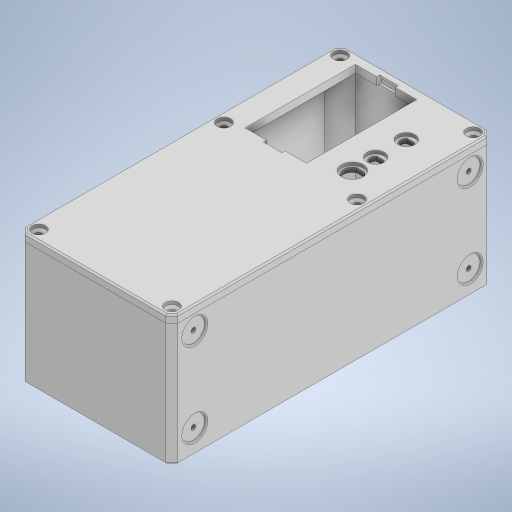
# Autodesk Inventor part: Light Beacon Box
Saved by Autodesk Inventor 2024 (Build 280153020, 153B)
## iProperties
Created: 2023-08-06
Part Number: Light Beacon Box
Material: Generic
Document SubType Name: Modeling
Designer: torban
Density: 1 g/cm^3
Appearance: Default
Author: torban
Autodesk Inventor part; units mm, degrees
ref_plane "YZ Plane" through (0, 0, 0) normal (1, 0, 0) x (0, 1, 0)
ref_plane "XZ Plane" through (0, 0, 0) normal (0, 1, 0) x (-1, 0, 0)
ref_plane "XY Plane" through (0, 0, 0) normal (0, 0, 1) x (1, 0, 0)
sketch "Sketch1" plane through (0, 0, 0) normal (0, 1, 0) x (-1, 0, 0)
  line L0 (0, 0) -> (90, 0)
  line L1 (90, 0) -> (90, -120)
  line L2 (90, -120) -> (0, -120)
  line L3 (0, -120) -> (0, 0)
  line L4 (90, -120) -> (0, -120)
  line L5 (0, -120) -> (0, -200)
  line L6 (0, -200) -> (90, -200)
  line L7 (90, -200) -> (90, -120)
  line L8 (95, -125) -> (95, 5)
  line L9 (95, 5) -> (-5, 5)
  line L10 (-5, 5) -> (-5, -125)
  line L11 (-5, -125) -> (95, -125)
  line L12 (95, -115) -> (-5, -115)
  line L13 (-5, -115) -> (-5, -205)
  line L14 (-5, -205) -> (95, -205)
  line L15 (95, -205) -> (95, -115)
  point P0 (0, -125)
  point P1 (90, -125)
  dimension "d0" = 120
  dimension "d1" = 90
  dimension "d2" = 90
  dimension "d3" = 80
  dimension "d4" = 5
  dimension "d5" = 5
  constraints: 32 end point, 8 parallel, 4 perpendicular, 2 horizontal, 6 other
  measures "d0" distance of L0.end L1.end
  measures "d1" distance of L1.end L2.end
  measures "d2" distance of L6.end L5.end
  measures "d3" distance of L6.end L1.end
  measures "d4" distance between parallel lines of L1 L8
  measures "d5" distance between parallel lines of L7 L15
extrude "Extrusion1" add sketch "Sketch1" along normal blind 75 contours L3 L12 L10 L9 L8 L1 L0 | L3 L5 L11 L10 L12 | L12 L8 L11 L7 L1 | L2 L7 L11 L5 | L5 L6 L7 L11 L15 L14 L13
sketch "Sketch3" plane through (0, 0, 0) normal (0, -1, 0) x (1, 0, 0)
  line L0 (0, -200) -> (0, -125) projected
  line L1 (0, -125) -> (-90, -125) projected
  line L2 (-90, -125) -> (-90, -200) projected
  line L3 (-90, -200) -> (0, -200) projected
  line L4 (-90, -120) -> (0, -120) projected
  line L5 (0, -120) -> (0, 0) projected
  line L6 (0, 0) -> (-90, 0) projected
  line L7 (-90, 0) -> (-90, -120) projected
  line L8 (-95, 5) -> (5, 5) projected
  line L9 (5, 5) -> (5, -205) projected
  line L10 (5, -205) -> (-95, -205) projected
  line L11 (-95, -205) -> (-95, 5) projected
extrude "Extrusion2" add sketch "Sketch3" along normal blind 5 contours L3 L2 L1 L0 | L7 L6 L5 L4 | L8 L9 L10 L11
sketch "Sketch4" plane through (-90, 75, -120) normal (0, 0, 1) x (1, 0, 0)
  line L0 (95, -80) -> (-5, -80) projected
  line L1 (-5, -80) -> (-5, 0) projected
  line L2 (-5, 0) -> (0, 0) projected
  line L3 (0, -75) -> (0, 0) projected
  line L4 (0, -75) -> (90, -75) projected
  line L5 (90, 0) -> (90, -75) projected
  line L6 (0, 0) -> (90, 0) projected
  line L7 (95, 0) -> (95, -80) projected
  line L8 (90, 0) -> (95, 0) projected
  line L9 (0, -55) -> (90, -55)
  line L10 (90, -75) -> (90, 0) projected
  line L11 (0, -55) -> (20, -55)
  line L12 (20, -55) -> (20, 0)
  line L13 (90, -55) -> (70, -55)
  line L14 (70, -55) -> (70, 0)
  circle A0 centre (20, -55) radius 5
  circle A1 centre (70, -55) radius 5
  dimension "d10" = 20
  dimension "d11" = 20
  dimension "d12" = 20
  dimension "d13" = 10
  dimension "d14" = 10
  constraints: 10 end point, 6 point on line, 3 perpendicular, 2 centre point, 2 coincident
  measures "d10" distance between parallel lines of L4 L9
  measures "d11" distance of L9.start L11.end
  measures "d12" distance of L9.end L13.end
  measures "d13" diameter of A0
  measures "d14" diameter of A1
extrude "Extrusion3" cut sketch "Sketch4" against normal up to surface (5 mm away) contours A1 L9 | L9 L14 A1 | L14 L9 A1 | A0 L12 L9 | L9 A0 | A0 L9 L12
chamfer "Chamfer1" distance 10 angle 45 8 edges at (-90, 37.5, -120) (-90, 37.5, -200) (-90, 37.5, 0) (0, 37.5, 0) (0, 37.5, -120) (0, 37.5, -200) (0, 37.5, -125) (-90, 37.5, -125)
sketch "Sketch5" plane through (0, 75, 0) normal (0, 1, 0) x (1, 0, 0)
  line L0 (-10, 125) -> (0, 135) projected
  line L1 (0, 135) -> (0, 190) projected
  line L2 (0, 190) -> (-10, 200) projected
  line L3 (-10, 200) -> (-80, 200) projected
  line L4 (-80, 200) -> (-90, 190) projected
  line L5 (-90, 190) -> (-90, 135) projected
  line L6 (-90, 135) -> (-80, 125) projected
  line L7 (-80, 125) -> (-10, 125) projected
  line L8 (-10, 0) -> (0, 10) projected
  line L9 (0, 10) -> (0, 110) projected
  line L10 (0, 110) -> (-10, 120) projected
  line L11 (-10, 120) -> (-80, 120) projected
  line L12 (-80, 120) -> (-90, 110) projected
  line L13 (-90, 110) -> (-90, 10) projected
  line L14 (-90, 10) -> (-80, 0) projected
  line L15 (-80, 0) -> (-10, 0) projected
  line L16 (5, -5) -> (-95, -5) projected
  line L17 (-95, -5) -> (-95, 205) projected
  line L18 (-95, 205) -> (5, 205) projected
  line L19 (5, 205) -> (5, -5) projected
  line L20 (-88.5, 198.5) -> (-88.5, 1.5)
  line L21 (-88.5, 1.5) -> (-1.5, 1.5)
  line L22 (-1.5, 1.5) -> (-1.5, 198.5)
  line L23 (-1.5, 198.5) -> (-88.5, 198.5)
  line L24 (-75, 120) -> (-75, 125) projected
  line L25 (-75, 122.5) -> (-88.5, 122.5)
  line L26 (-75, 122.5) -> (-1.5, 122.5)
  point P0 (0, 0)
  dimension "d20" = 6.5
  dimension "d80" = 0
  constraints: 12 end point, 5 coincident, 4 point on line, 1 perpendicular, 6 other
  measures "d20" distance between parallel lines of L17 L20
  measures "d80" distance from line of L23 point (-1.5, 198.5)
hole "Hole1" at (-88.5, 75, -1.5) at (-88.5, 75, -198.5) at (-1.5, 75, -198.5) at (-1.5, 75, -1.5) at (-88.5, 75, -122.5) at (-1.5, 75, -122.5) direction (0, -1, 0) diameter 4.69 depth 20 tip angle 118
chamfer "Chamfer2" distance 4 angle 45 4 edges at (-95, 35, 5) (5, 35, 5) (-95, 35, -205) (5, 35, -205)
sketch "Sketch6" plane through (0, 75, 0) normal (0, 1, 0) x (1, 0, 0)
  line L0 (-91, -5) -> (-95, -1) projected
  line L1 (-95, -1) -> (-95, 201) projected
  line L2 (-95, 201) -> (-91, 205) projected
  line L3 (-91, 205) -> (1, 205) projected
  line L4 (1, 205) -> (5, 201) projected
  line L5 (5, 201) -> (5, -1) projected
  line L6 (5, -1) -> (1, -5) projected
  line L7 (1, -5) -> (-91, -5) projected
  line L8 (-80, 125) -> (-10, 125) projected
  line L9 (-10, 125) -> (0, 135) projected
  line L10 (0, 135) -> (0, 190) projected
  line L11 (0, 190) -> (-10, 200) projected
  line L12 (-10, 200) -> (-80, 200) projected
  line L13 (-80, 200) -> (-90, 190) projected
  line L14 (-90, 190) -> (-90, 135) projected
  line L15 (-90, 135) -> (-80, 125) projected
  line L16 (0, 10) -> (0, 110) projected
  line L17 (0, 110) -> (-10, 120) projected
  line L18 (-10, 120) -> (-80, 120) projected
  line L19 (-80, 120) -> (-90, 110) projected
  line L20 (-90, 110) -> (-90, 10) projected
  line L21 (-90, 10) -> (-80, 0) projected
  line L22 (-80, 0) -> (-10, 0) projected
  line L23 (-10, 0) -> (0, 10) projected
  circle A0 centre (-88.5, 1.5) radius 2.345 projected
  circle A1 centre (-88.5, 198.5) radius 2.345 projected
  circle A2 centre (-1.5, 198.5) radius 2.345 projected
  circle A3 centre (-1.5, 1.5) radius 2.345 projected
  circle A4 centre (-88.5, 122.5) radius 2.345 projected
  circle A5 centre (-1.5, 122.5) radius 2.345 projected
  point P0 (0, 0)
extrude "Extrusion4" add sketch "Sketch6" along normal blind 5 separate body
sketch "Sketch7" plane through (0, 80, 0) normal (0, 1, 0) x (1, 0, 0)
  line L0 (-80, 125) -> (-10, 125) projected
  line L1 (-10, 125) -> (0, 135) projected
  line L2 (0, 135) -> (0, 190) projected
  line L3 (0, 190) -> (-10, 200) projected
  line L4 (-10, 200) -> (-80, 200) projected
  line L5 (-80, 200) -> (-90, 190) projected
  line L6 (-90, 190) -> (-90, 135) projected
  line L7 (-90, 135) -> (-80, 125) projected
  line L8 (0, 10) -> (0, 110) projected
  line L9 (0, 110) -> (-10, 120) projected
  line L10 (-10, 120) -> (-80, 120) projected
  line L11 (-80, 120) -> (-90, 110) projected
  line L12 (-90, 110) -> (-90, 10) projected
  line L13 (-90, 10) -> (-80, 0) projected
  line L14 (-80, 0) -> (-10, 0) projected
  line L15 (-10, 0) -> (0, 10) projected
  circle A0 centre (-88.5, 1.5) radius 2.345 projected
  circle A1 centre (-88.5, 198.5) radius 2.345 projected
  circle A2 centre (-1.5, 198.5) radius 2.345 projected
  circle A3 centre (-1.5, 1.5) radius 2.345 projected
  circle A4 centre (-1.5, 122.5) radius 2.345 projected
  circle A5 centre (-88.5, 122.5) radius 2.345 projected
  line L16 (1, -5) -> (-91, -5) projected
  line L17 (-91, -5) -> (-95, -1) projected
  line L18 (-95, -1) -> (-95, 201) projected
  line L19 (-95, 201) -> (-91, 205) projected
  line L20 (-91, 205) -> (1, 205) projected
  line L21 (1, 205) -> (5, 201) projected
  line L22 (5, 201) -> (5, -1) projected
  line L23 (5, -1) -> (1, -5) projected
  line L24 (-78.5, 126.5) -> (-38.5, 126.5)
  line L25 (-38.5, 126.5) -> (-38.5, 198.5)
  line L26 (-38.5, 198.5) -> (-78.5, 198.5)
  line L27 (-78.5, 198.5) -> (-78.5, 126.5)
  point P0 (0, 0)
  point P1 (-58.5, 198.5)
  dimension "d33" = 72
  dimension "d35" = 40
  dimension "d40" = 1.5
  dimension "d41" = 1.5
  constraints: 8 end point, 2 parallel, 1 horizontal, 1 midpoint, 1 perpendicular
  measures "d33" distance between parallel lines of L26 L24
  measures "d35" distance of L25.end L26.end
  measures "d40" distance from line of L4.end L27
  measures "d41" distance between parallel lines of L0 L24
extrude "Extrusion5" add sketch "Sketch7" against normal blind 5 contours L7 L6 L5 L4 L3 L2 L1 L0 | L15 L14 L13 L12 L11 L10 L9 L8 | L16 L17 L18 L19 L20 L21 L22 L23 bodies 2
sketch "Sketch8" plane through (0, 80, 0) normal (0, 1, 0) x (1, 0, 0)
  line L0 (-38.5, 198.5) -> (-78.5, 198.5) projected
  line L1 (-78.5, 198.5) -> (-78.5, 126.5) projected
  line L2 (-78.5, 126.5) -> (-38.5, 126.5) projected
  line L3 (-38.5, 126.5) -> (-38.5, 198.5) projected
  circle A0 centre (-88.5, 1.5) radius 2.345 projected
  circle A1 centre (-88.5, 198.5) radius 2.345 projected
  circle A2 centre (-1.5, 198.5) radius 2.345 projected
  circle A3 centre (-1.5, 1.5) radius 2.345 projected
  circle A4 centre (-1.5, 122.5) radius 2.345 projected
  circle A5 centre (-88.5, 122.5) radius 2.345 projected
  line L4 (1, -5) -> (-91, -5) projected
  line L5 (-91, -5) -> (-95, -1) projected
  line L6 (-95, -1) -> (-95, 201) projected
  line L7 (-95, 201) -> (-91, 205) projected
  line L8 (-91, 205) -> (1, 205) projected
  line L9 (1, 205) -> (5, 201) projected
  line L10 (5, 201) -> (5, -1) projected
  line L11 (5, -1) -> (1, -5) projected
  line L12 (-64.5, 124.5) -> (-52.5, 124.5)
  line L13 (-52.5, 124.5) -> (-52.5, 200.5)
  line L14 (-52.5, 200.5) -> (-64.5, 200.5)
  line L15 (-64.5, 200.5) -> (-64.5, 124.5)
  point P0 (0, 0)
  point P1 (-64.5, 198.5)
  point P2 (-52.5, 198.5)
  point P3 (-52.5, 126.5)
  point P4 (-64.5, 126.5)
  dimension "d44" = 12
  dimension "d46" = 14
  dimension "d47" = 14
  dimension "d48" = 76
  dimension "d49" = 2
  constraints: 8 end point, 2 parallel, 1 horizontal, 1 perpendicular
  measures "d44" distance of L12.start L12.end
  measures "d46" distance between parallel lines of L3 L13
  measures "d47" distance between parallel lines of L1 L15
  measures "d48" distance between parallel lines of L14 L12
  measures "d49" distance between parallel lines of L2 L12
extrude "Extrusion6" cut sketch "Sketch8" against normal blind 5 contours L0 L15 L14 L13 | L13 L12 L15 L2 bodies 2
sketch "Sketch9" plane through (0, 75, 0) normal (0, 1, 0) x (1, 0, 0)
  line L0 (-91, -5) -> (-95, -1) projected
  line L1 (-95, -1) -> (-95, 201) projected
  line L2 (-95, 201) -> (-91, 205) projected
  line L3 (-91, 205) -> (1, 205) projected
  line L4 (1, 205) -> (5, 201) projected
  line L5 (5, 201) -> (5, -1) projected
  line L6 (5, -1) -> (1, -5) projected
  line L7 (1, -5) -> (-91, -5) projected
  line L8 (-80, 125) -> (-10, 125) projected
  line L9 (-10, 125) -> (0, 135) projected
  line L10 (0, 135) -> (0, 190) projected
  line L11 (0, 190) -> (-10, 200) projected
  line L12 (-10, 200) -> (-80, 200) projected
  line L13 (-80, 200) -> (-90, 190) projected
  line L14 (-90, 190) -> (-90, 135) projected
  line L15 (-90, 135) -> (-80, 125) projected
  line L16 (0, 10) -> (0, 110) projected
  line L17 (0, 110) -> (-10, 120) projected
  line L18 (-10, 120) -> (-80, 120) projected
  line L19 (-80, 120) -> (-90, 110) projected
  line L20 (-90, 110) -> (-90, 10) projected
  line L21 (-90, 10) -> (-80, 0) projected
  line L22 (-80, 0) -> (-10, 0) projected
  line L23 (-10, 0) -> (0, 10) projected
  circle A0 centre (-88.5, 1.5) radius 2.345 projected
  circle A1 centre (-88.5, 198.5) radius 2.345 projected
  circle A2 centre (-1.5, 198.5) radius 2.345 projected
  circle A3 centre (-1.5, 1.5) radius 2.345 projected
  circle A4 centre (-88.5, 122.5) radius 2.345 projected
  circle A5 centre (-1.5, 122.5) radius 2.345 projected
  line L24 (-64.5, 126.5) -> (-64.5, 124.5) projected
  line L25 (-64.5, 124.5) -> (-52.5, 124.5) projected
  line L26 (-52.5, 124.5) -> (-52.5, 126.5) projected
  line L27 (-52.5, 126.5) -> (-38.5, 126.5) projected
  line L28 (-38.5, 126.5) -> (-38.5, 198.5) projected
  line L29 (-38.5, 198.5) -> (-52.5, 198.5) projected
  line L30 (-52.5, 198.5) -> (-52.5, 200.5) projected
  line L31 (-52.5, 200.5) -> (-64.5, 200.5) projected
  line L32 (-64.5, 200.5) -> (-64.5, 198.5) projected
  line L33 (-64.5, 198.5) -> (-78.5, 198.5) projected
  line L34 (-78.5, 198.5) -> (-78.5, 126.5) projected
  line L35 (-78.5, 126.5) -> (-64.5, 126.5) projected
  circle A6 centre (-88.5, 1.5) radius 2.345 projected
  circle A7 centre (-88.5, 198.5) radius 2.345 projected
  circle A8 centre (-1.5, 198.5) radius 2.345 projected
  circle A9 centre (-1.5, 1.5) radius 2.345 projected
  circle A10 centre (-1.5, 122.5) radius 2.345 projected
  circle A11 centre (-88.5, 122.5) radius 2.345 projected
  line L36 (5, -1) -> (1, -5) projected
  line L37 (1, -5) -> (-91, -5) projected
  line L38 (-91, -5) -> (-95, -1) projected
  line L39 (-95, -1) -> (-95, 201) projected
  line L40 (-95, 201) -> (-91, 205) projected
  line L41 (-91, 205) -> (1, 205) projected
  line L42 (1, 205) -> (5, 201) projected
  line L43 (5, 201) -> (5, -1) projected
  line L44 (-64.5, 126.5) -> (-52.5, 126.5)
  line L45 (-52.5, 126.5) -> (-52.5, 123.5)
  line L46 (-52.5, 123.5) -> (-64.5, 123.5)
  line L47 (-64.5, 123.5) -> (-64.5, 126.5)
  line L48 (-64.5, 198.5) -> (-52.5, 198.5)
  line L49 (-52.5, 198.5) -> (-52.5, 201.5)
  line L50 (-52.5, 201.5) -> (-64.5, 201.5)
  line L51 (-64.5, 201.5) -> (-64.5, 198.5)
  point P0 (0, 0)
  point P1 (-52.5, 199.5)
  point P2 (-52.5, 200)
  dimension "d52" = 78
  dimension "d53" = 1
  dimension "d54" = 1
  dimension "d55" = 0
  dimension "d56" = 0
  constraints: 16 end point, 4 parallel, 4 point on line, 2 horizontal, 2 midpoint, 2 perpendicular
  measures "d52" distance between parallel lines of L50 L46
  measures "d53" distance between parallel lines of L25 L46
  measures "d54" distance between parallel lines of L50 L31
  measures "d55" distance between parallel lines of L32 L51
  measures "d56" horizontal distance of point (-52.5, 199.5) point (-52.5, 200)
extrude "Extrusion7" cut sketch "Sketch9" along normal blind 3.5 contours L25 L45 L46 L47 | L51 L50 L49 L31 bodies 2
sketch "Sketch10" plane through (0, 80, 0) normal (0, 1, 0) x (1, 0, 0)
  line L0 (-52.5, 200.5) -> (-52.5, 198.5) projected
  line L1 (-52.5, 198.5) -> (-38.5, 198.5) projected
  line L2 (-38.5, 198.5) -> (-38.5, 126.5) projected
  line L3 (-38.5, 126.5) -> (-52.5, 126.5) projected
  line L4 (-52.5, 126.5) -> (-52.5, 124.5) projected
  line L5 (-52.5, 124.5) -> (-64.5, 124.5) projected
  line L6 (-64.5, 124.5) -> (-64.5, 126.5) projected
  line L7 (-64.5, 126.5) -> (-78.5, 126.5) projected
  line L8 (-78.5, 126.5) -> (-78.5, 198.5) projected
  line L9 (-78.5, 198.5) -> (-64.5, 198.5) projected
  line L10 (-64.5, 198.5) -> (-64.5, 200.5) projected
  line L11 (-64.5, 200.5) -> (-52.5, 200.5) projected
  line L12 (1, -5) -> (5, -1) projected
  line L13 (5, -1) -> (5, 201) projected
  line L14 (5, 201) -> (1, 205) projected
  line L15 (1, 205) -> (-91, 205) projected
  line L16 (-91, 205) -> (-95, 201) projected
  line L17 (-95, 201) -> (-95, -1) projected
  line L18 (-95, -1) -> (-91, -5) projected
  line L19 (-91, -5) -> (1, -5) projected
  circle A0 centre (-88.5, 122.5) radius 2.345 projected
  circle A1 centre (-1.5, 122.5) radius 2.345 projected
  circle A2 centre (-1.5, 1.5) radius 2.345 projected
  circle A3 centre (-1.5, 198.5) radius 2.345 projected
  circle A4 centre (-88.5, 198.5) radius 2.345 projected
  circle A5 centre (-88.5, 1.5) radius 2.345 projected
  line L20 (0, 190) -> (0, 135) projected
  line L21 (-38.5, 126.5) -> (-38.5, 198.5) projected
  line L22 (-38.5, 162.5) -> (0, 162.5)
  line L23 (-19.25, 162.5) -> (-19.25, 172.5)
  line L24 (-19.25, 172.5) -> (-19.25, 152.5)
  circle A6 centre (-19.25, 172.5) radius 3.875
  circle A7 centre (-19.25, 152.5) radius 3.875
  line L25 (-21.7027, 149.5) -> (-16.7973, 149.5)
  line L26 (-16.7973, 149.5) -> (-16.7973, 155.5)
  line L27 (-16.7973, 155.5) -> (-21.7027, 155.5)
  line L28 (-21.7027, 155.5) -> (-21.7027, 149.5)
  line L29 (-21.7027, 149.5) -> (-16.7973, 155.5) construction
  line L30 (-16.7973, 149.5) -> (-21.7027, 155.5) construction
  line L31 (-21.7027, 175.5) -> (-16.7973, 175.5)
  line L32 (-16.7973, 175.5) -> (-16.7973, 169.5)
  line L33 (-16.7973, 169.5) -> (-21.7027, 169.5)
  line L34 (-21.7027, 169.5) -> (-21.7027, 175.5)
  line L35 (-21.7027, 175.5) -> (-16.7973, 169.5) construction
  line L36 (-16.7973, 175.5) -> (-21.7027, 169.5) construction
  point P0 (0, 0)
  dimension "d61" = 7.75
  dimension "d62" = 7.75
  dimension "d59" = 10
  dimension "d60" = 20
  dimension "d63" = 6
  constraints: 30 end point, 7 midpoint, 4 parallel, 3 perpendicular, 2 coincident, 2 horizontal, 2 point on line, 6 other
  measures "d59" distance of L23.start L23.end
  measures "d60" distance of L23.end L24.end
  measures "d63" distance of L26.end L25.end
extrude "Extrusion8" cut sketch "Sketch10" against normal blind 5 contours L33 L34 L31 L32 | A6 L34 | L32 A6 | L27 L26 L25 L28 | A7 L26 | L28 A7 bodies 2
sketch "Sketch11" plane through (0, 80, 0) normal (0, 1, 0) x (1, 0, 0)
  arc A0 (-16.7973, 169.5) -> (-16.7973, 175.5) centre (-19.25, 172.5) ccw projected
  line L0 (-16.7973, 169.5) -> (-21.7027, 169.5) projected
  arc A1 (-21.7027, 175.5) -> (-21.7027, 169.5) centre (-19.25, 172.5) ccw projected
  line L1 (-21.7027, 175.5) -> (-16.7973, 175.5) projected
  arc A2 (-16.7973, 149.5) -> (-16.7973, 155.5) centre (-19.25, 152.5) ccw projected
  line L2 (-16.7973, 149.5) -> (-21.7027, 149.5) projected
  arc A3 (-21.7027, 155.5) -> (-21.7027, 149.5) centre (-19.25, 152.5) ccw projected
  line L3 (-21.7027, 155.5) -> (-16.7973, 155.5) projected
  line L4 (-52.5, 200.5) -> (-52.5, 198.5) projected
  line L5 (-52.5, 198.5) -> (-38.5, 198.5) projected
  line L6 (-38.5, 198.5) -> (-38.5, 126.5) projected
  line L7 (-38.5, 126.5) -> (-52.5, 126.5) projected
  line L8 (-52.5, 126.5) -> (-52.5, 124.5) projected
  line L9 (-52.5, 124.5) -> (-64.5, 124.5) projected
  line L10 (-64.5, 124.5) -> (-64.5, 126.5) projected
  line L11 (-64.5, 126.5) -> (-78.5, 126.5) projected
  line L12 (-78.5, 126.5) -> (-78.5, 198.5) projected
  line L13 (-78.5, 198.5) -> (-64.5, 198.5) projected
  line L14 (-64.5, 198.5) -> (-64.5, 200.5) projected
  line L15 (-64.5, 200.5) -> (-52.5, 200.5) projected
  line L16 (1, -5) -> (5, -1) projected
  line L17 (5, -1) -> (5, 201) projected
  line L18 (5, 201) -> (1, 205) projected
  line L19 (1, 205) -> (-91, 205) projected
  line L20 (-91, 205) -> (-95, 201) projected
  line L21 (-95, 201) -> (-95, -1) projected
  line L22 (-95, -1) -> (-91, -5) projected
  line L23 (-91, -5) -> (1, -5) projected
  circle A4 centre (-88.5, 122.5) radius 2.345 projected
  circle A5 centre (-1.5, 122.5) radius 2.345 projected
  circle A6 centre (-1.5, 1.5) radius 2.345 projected
  circle A7 centre (-1.5, 198.5) radius 2.345 projected
  circle A8 centre (-88.5, 198.5) radius 2.345 projected
  circle A9 centre (-88.5, 1.5) radius 2.345 projected
  point P0 (0, 0)
  point P1 (-1.5, 1.5)
  constraints: 5 coincident
hole "Hole3" at (-88.5, 80, -1.5) at (-88.5, 80, -122.5) at (-88.5, 80, -198.5) at (-1.5, 80, -198.5) at (-1.5, 80, -122.5) at (-1.5, 80, -1.5) direction (0, -1, 0) diameter 8.7 depth 2 tip angle 118 bodies 2
sketch "Sketch2" plane through (0, 0, -125) normal (0, 0, -1) x (-1, 0, 0)
  line L0 (-5, -5) -> (-5, 75) projected
  line L1 (-5, 75) -> (10, 75) projected
  line L2 (80, 75) -> (95, 75) projected
  line L3 (95, 75) -> (95, -5) projected
  line L4 (80, 0) -> (80, 75) projected
  line L5 (10, 75) -> (80, 75) projected
  line L6 (95, -5) -> (-5, -5) projected
  circle A0 centre (20, 20) radius 5 projected
  circle A1 centre (70, 20) radius 5 projected
  line L7 (95, 75) -> (64.5, 75) projected
  line L8 (64.5, 75) -> (64.5, 80) projected
  line L9 (64.5, 80) -> (84.9402, 80) projected
  line L10 (84.9402, 80) -> (84.9402, 78) projected
  line L11 (92.0598, 78) -> (92.0598, 80) projected
  line L12 (92.0598, 80) -> (95, 80) projected
  line L13 (95, 80) -> (95, 75) projected
  line L14 (52.5, 75) -> (-5, 75) projected
  line L15 (-5, 75) -> (-5, 80) projected
  line L16 (-5, 80) -> (-2.0598, 80) projected
  line L17 (-2.0598, 80) -> (-2.0598, 78) projected
  line L18 (5.0598, 78) -> (5.0598, 80) projected
  line L19 (5.0598, 80) -> (52.5, 80) projected
  line L20 (52.5, 80) -> (52.5, 75) projected
  line L21 (10, 0) -> (10, 75) projected
  line L22 (10, 0) -> (80, 0) projected
  constraints: 2 horizontal alignment
sketch "Sketch12" plane through (0, 80, 0) normal (0, 1, 0) x (1, 0, 0)
  line L0 (-90, 10) -> (-90, 110) projected
  circle A0 centre (-88.5, 1.5) radius 4.35 projected
  line L1 (-90, 10) -> (-80, 0) projected
  line L2 (-10, 0) -> (-80, 0) projected
  line L3 (-10, 0) -> (0, 10) projected
  line L4 (-38.5, 198.5) -> (-38.5, 126.5) projected
  line L5 (-38.5, 162.5) -> (0, 162.5)
  line L6 (0, 190) -> (0, 135) projected
  line L7 (-10, 125) -> (-80, 125) projected
  line L8 (-10, 125) -> (-80, 125) projected
  line L9 (-21.7027, 149.5) -> (-16.7973, 149.5) projected
  line L10 (-19.25, 149.5) -> (-19.25, 125)
  circle A1 centre (-19.25, 137.25) radius 5.8
  line L11 (-16.7847, 142.5) -> (-21.7153, 142.5)
  line L12 (-21.7153, 142.5) -> (-21.7153, 132)
  line L13 (-21.7153, 132) -> (-16.7847, 132)
  line L14 (-16.7847, 132) -> (-16.7847, 142.5)
  line L15 (-16.7847, 142.5) -> (-21.7153, 132) construction
  line L16 (-21.7153, 142.5) -> (-16.7847, 132) construction
  point P0 (0, 0)
  point P1 (-10, 120)
  dimension "d84" = 11.6
  dimension "d85" = 10.5
  constraints: 16 end point, 6 midpoint, 2 parallel, 2 perpendicular, 1 horizontal, 1 point on line, 3 other
  measures "d85" distance of L12.end L11.end
extrude "Extrusion9" cut sketch "Sketch12" against normal blind 5 contours L11 L14 L13 L10 | L10 L13 L12 L11 | A1 L14 | L12 A1 bodies 2
fillet "Fillet1" radius 2.5 4 edges at (-75, 20, -120) (-75, 20, -125) (-25, 20, -120) (-25, 20, -125)
sketch "Sketch13" plane through (0, 80, 0) normal (0, 1, 0) x (1, 0, 0)
  arc A0 (-21.7153, 142.5) -> (-21.7153, 132) centre (-19.25, 137.25) ccw projected
  line L0 (-21.7153, 142.5) -> (-16.7847, 142.5) projected
  arc A1 (-16.7847, 132) -> (-16.7847, 142.5) centre (-19.25, 137.25) ccw projected
  line L1 (-16.7847, 132) -> (-21.7153, 132) projected
  circle A2 centre (-1.5, 1.5) radius 4.35 projected
  circle A3 centre (-1.5, 122.5) radius 4.35 projected
  circle A4 centre (-1.5, 198.5) radius 4.35 projected
  circle A5 centre (-88.5, 198.5) radius 4.35 projected
  circle A6 centre (-88.5, 122.5) radius 4.35 projected
  circle A7 centre (-88.5, 1.5) radius 4.35 projected
  arc A8 (-16.7973, 169.5) -> (-16.7973, 175.5) centre (-19.25, 172.5) ccw projected
  line L2 (-16.7973, 169.5) -> (-21.7027, 169.5) projected
  arc A9 (-21.7027, 175.5) -> (-21.7027, 169.5) centre (-19.25, 172.5) ccw projected
  line L3 (-21.7027, 175.5) -> (-16.7973, 175.5) projected
  arc A10 (-16.7973, 149.5) -> (-16.7973, 155.5) centre (-19.25, 152.5) ccw projected
  line L4 (-16.7973, 149.5) -> (-21.7027, 149.5) projected
  arc A11 (-21.7027, 155.5) -> (-21.7027, 149.5) centre (-19.25, 152.5) ccw projected
  line L5 (-21.7027, 155.5) -> (-16.7973, 155.5) projected
  line L6 (-52.5, 200.5) -> (-52.5, 198.5) projected
  line L7 (-52.5, 198.5) -> (-38.5, 198.5) projected
  line L8 (-38.5, 198.5) -> (-38.5, 126.5) projected
  line L9 (-38.5, 126.5) -> (-52.5, 126.5) projected
  line L10 (-52.5, 126.5) -> (-52.5, 124.5) projected
  line L11 (-52.5, 124.5) -> (-64.5, 124.5) projected
  line L12 (-64.5, 124.5) -> (-64.5, 126.5) projected
  line L13 (-64.5, 126.5) -> (-78.5, 126.5) projected
  line L14 (-78.5, 126.5) -> (-78.5, 198.5) projected
  line L15 (-78.5, 198.5) -> (-64.5, 198.5) projected
  line L16 (-64.5, 198.5) -> (-64.5, 200.5) projected
  line L17 (-64.5, 200.5) -> (-52.5, 200.5) projected
  line L18 (1, -5) -> (5, -1) projected
  line L19 (5, -1) -> (5, 201) projected
  line L20 (5, 201) -> (1, 205) projected
  line L21 (1, 205) -> (-91, 205) projected
  line L22 (-91, 205) -> (-95, 201) projected
  line L23 (-95, 201) -> (-95, -1) projected
  line L24 (-95, -1) -> (-91, -5) projected
  line L25 (-91, -5) -> (1, -5) projected
  circle A12 centre (-19.25, 137.25) radius 7
  circle A13 centre (-19.25, 152.5) radius 5.6
  circle A14 centre (-19.25, 172.5) radius 5.6
  point P0 (0, 0)
  dimension "d89" = 14
  dimension "d92" = 11.2
  dimension "d93" = 11.2
  constraints: 3 centre point, 3 coincident
  measures "d89" diameter of A12
  measures "d92" diameter of A13
  measures "d93" diameter of A14
extrude "Extrusion10" cut sketch "Sketch13" against normal blind 2 contours A12 | A13 | A14 bodies 2
sketch "Sketch14" plane through (5, -5, -201) normal (1, 0, 0) x (0, 0, -1)
  line L0 (-206, 85) -> (-202, 85) projected
  line L1 (4, 0) -> (0, 0) projected
  line L2 (-206, 85) -> (4, 85)
  line L3 (4, 85) -> (4, 0)
  line L4 (4, 0) -> (-206, 0)
  line L5 (-206, 0) -> (-206, 85)
  line L6 (-11, 70) -> (-191, 70)
  line L7 (-191, 70) -> (-191, 15)
  line L8 (-191, 15) -> (-11, 15)
  line L9 (-11, 15) -> (-11, 70)
  circle A0 centre (-191, 70) radius 7.5
  circle A1 centre (-191, 15) radius 7.5
  circle A2 centre (-11, 70) radius 7.5
  circle A3 centre (-11, 15) radius 7.5
  point P0 (-201, 5)
  dimension "d94" = 15
  dimension "d95" = 15
  dimension "d96" = 15
  dimension "d97" = 15
  dimension "d98" = 15
  constraints: 16 end point, 4 centre point, 4 coincident, 4 parallel, 2 perpendicular, 1 horizontal, 3 other
  measures "d94" distance between parallel lines of L2 L6
  measures "d95" diameter of A0
  measures "d96" diameter of A1
  measures "d97" diameter of A2
  measures "d98" diameter of A3
extrude "Extrusion11" cut sketch "Sketch14" against normal blind 1 contours A0 L7 L6 | L6 L7 A0 | A2 L9 L6 | L6 L9 A2 | A1 L8 L7 | L7 L8 A1 | A3 L8 L9 | L9 L8 A3 bodies 1
fillet "Fillet2" radius 1 4 edges at (5, 65, -2.5) (5, 10, -2.5) (5, 10, -182.5) (5, 65, -182.5)
sketch "Sketch15" plane through (5, -5, -201) normal (1, 0, 0) x (0, 0, -1)
  circle A0 centre (-11, 70) radius 8.5 projected
  circle A1 centre (-11, 15) radius 8.5 projected
  circle A2 centre (-191, 70) radius 8.5 projected
  line L0 (0, 80) -> (0, 0) projected
  line L1 (0, 0) -> (-202, 0) projected
  line L2 (-202, 0) -> (-202, 80) projected
  line L3 (-202, 80) -> (0, 80) projected
  circle A3 centre (-191, 15) radius 8.5 projected
  line L4 (0, 80) -> (-202, 80) projected
  line L5 (-202, 80) -> (-202, 85) projected
  line L6 (-202, 85) -> (0, 85) projected
  line L7 (0, 85) -> (0, 80) projected
  point P0 (-201, 5)
  constraints: 4 coincident
hole "Hole4" at (5, 65, -10) at (5, 10, -10) at (5, 10, -190) at (5, 65, -190) direction (-1, 0, 0) diameter 3 depth 5 tip angle 118 bodies 1
sketch "Sketch16" plane through (0, 0, -190) normal (-1, 0, 0) x (0, 0, 1)
  line L0 (-6.6975, 55) -> (-6.6975, 75) projected
  line L1 (-6.6975, 75) -> (0, 75) projected
  line L2 (0, 66.5) -> (0, 75) projected
  arc A0 (0, 63.5) -> (0, 66.5) centre (0, 65) ccw projected
  line L3 (0, 11.5) -> (0, 63.5) projected
  arc A1 (0, 8.5) -> (0, 11.5) centre (0, 10) ccw projected
  line L4 (0, 0) -> (0, 8.5) projected
  line L5 (55, 0) -> (0, 0) projected
  line L6 (55, 75) -> (55, 0) projected
  line L7 (55, 75) -> (65.6975, 75) projected
  line L8 (65.6975, 75) -> (65.6975, 55) projected
  line L9 (69.3025, 55) -> (69.3025, 75) projected
  line L10 (69.3025, 75) -> (80, 75) projected
  line L11 (80, 0) -> (80, 75) projected
  line L12 (180, 0) -> (80, 0) projected
  line L13 (180, 8.5) -> (180, 0) projected
  arc A2 (180, 11.5) -> (180, 8.5) centre (180, 10) ccw projected
  line L14 (180, 63.5) -> (180, 11.5) projected
  arc A3 (180, 63.5) -> (180, 66.5) centre (180, 65) ccw projected
  line L15 (180, 75) -> (180, 66.5) projected
  line L16 (180, 75) -> (186.6975, 75) projected
  line L17 (186.6975, 75) -> (186.6975, 55) projected
  line L18 (190.3025, 55) -> (190.3025, 75) projected
  line L19 (190.3025, 75) -> (195, 75) projected
  line L20 (195, 75) -> (195, -5) projected
  line L21 (195, -5) -> (-15, -5) projected
  line L22 (-15, -5) -> (-15, 75) projected
  line L23 (-15, 75) -> (-10.3025, 75) projected
  line L24 (-10.3025, 75) -> (-10.3025, 55) projected
  line L25 (0, 75) -> (55, 75) projected
  arc A4 (0, 66.5) -> (0, 63.5) centre (0, 65) ccw projected
  arc A5 (0, 11.5) -> (0, 8.5) centre (0, 10) ccw projected
  line L26 (80, 75) -> (180, 75) projected
  arc A6 (180, 8.5) -> (180, 11.5) centre (180, 10) ccw projected
  arc A7 (180, 66.5) -> (180, 63.5) centre (180, 65) ccw projected
  line L27 (195, 75) -> (190.3025, 75) projected
  line L28 (190.3025, 75) -> (190.3025, 76.7953) projected
  line L29 (192.5832, 78) -> (192.5832, 80) projected
  line L30 (192.5832, 80) -> (195, 80) projected
  line L31 (195, 80) -> (195, 75) projected
  line L32 (186.6975, 75) -> (69.3025, 75) projected
  line L33 (69.3025, 75) -> (69.3025, 76.7953) projected
  line L34 (71.5832, 78) -> (71.5832, 80) projected
  line L35 (71.5832, 80) -> (184.4168, 80) projected
  line L36 (184.4168, 80) -> (184.4168, 78) projected
  line L37 (186.6975, 76.7953) -> (186.6975, 75) projected
  line L38 (65.6975, 75) -> (-6.6975, 75) projected
  line L39 (-6.6975, 75) -> (-6.6975, 76.7953) projected
  line L40 (-4.4168, 78) -> (-4.4168, 80) projected
  line L41 (-4.4168, 80) -> (63.4168, 80) projected
  line L42 (63.4168, 80) -> (63.4168, 78) projected
  line L43 (65.6975, 76.7953) -> (65.6975, 75) projected
  line L44 (-10.3025, 75) -> (-15, 75) projected
  line L45 (-15, 75) -> (-15, 80) projected
  line L46 (-15, 80) -> (-12.5832, 80) projected
  line L47 (-12.5832, 80) -> (-12.5832, 78) projected
  line L48 (-10.3025, 76.7953) -> (-10.3025, 75) projected
  circle A8 centre (180, 10) radius 7.5 projected
  circle A9 centre (180, 10) radius 4
  circle A10 centre (0, 10) radius 1.5 projected
  circle A11 centre (0, 10) radius 4
  circle A12 centre (0, 65) radius 4
  circle A13 centre (180, 65) radius 4
  point P0 (190, 0)
  point P1 (180, 6)
  point P2 (180, 14)
  point P3 (180, 61)
  point P4 (180, 69)
  point P5 (0, 69)
  point P6 (0, 61)
  point P7 (0, 14)
  point P8 (0, 6)
  dimension "d109" = 8
  dimension "d110" = 8
  dimension "d111" = 8
  dimension "d112" = 8
  constraints: 4 centre point, 4 coincident, 3 horizontal alignment, 6 other
  measures "d109" diameter of A9
  measures "d110" diameter of A11
  measures "d111" diameter of A12
  measures "d112" diameter of A13
extrude "Extrusion12" cut sketch "Sketch16" along normal blind 5 contours A4 L3 A12 L2 | A0 A4 | L3 A5 L4 A11 | A1 A5 | A13 L14 A3 L15 | L13 A6 L14 A9 | A3 A7 | A2 A6 bodies 1
chamfer "Chamfer3" distance 3.99 angle 45 4 edges at (-4, 10, -194) (-4, 65, -194) (-4, 65, -6) (-4, 10, -6)
chamfer "Chamfer4" distance 1 angle 45 16 edges at (-93, -5, -203) (-95, -5, -100) (-93, -5, 3) (-45, -5, -205) (5, -5, -100) (3, -5, -203) (3, -5, 3) (-45, -5, 5) (-93, 80, 3) (-95, 80, -100) (-45, 80, 5) (3, 80, 3) (5, 80, -100) (3, 80, -203) (-45, 80, -205) (-93, 80, -203)
equation "\"d47\" = d46"
equation "\"d96\" = d95"
equation "\"d97\" = d95"
equation "\"d98\" = d97"
body "Solid1"
